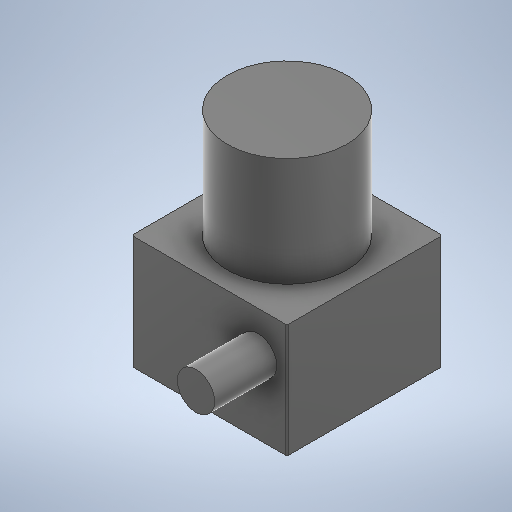
# Autodesk Inventor part: RE38S-600Z-1M-no-end
Saved by Autodesk Inventor 2026.2 (Build 302298010, 298A)
## iProperties
Created: 2026-05-12
Part Number: RE38S-600Z-1M-no-end
Material: ABS Plastic
Document SubType Name: Modeling
Designer: chanh
Density: 1.06 g/cm^3
Appearance: Smooth - White
Author: chanh
Autodesk Inventor part; units mm, degrees
ref_plane "YZ Plane" through (0, 0, 0) normal (1, 0, 0) x (0, 1, 0)
ref_plane "XZ Plane" through (0, 0, 0) normal (0, 1, 0) x (-1, 0, 0)
sketch "Sketch1" plane through (0, 0, 0) normal (0, 1, 0) x (-1, 0, 0)
  line L0 (-25, 25) -> (25, 25)
  line L1 (25, 25) -> (25, -25)
  line L2 (25, -25) -> (-25, -25)
  line L3 (-25, -25) -> (-25, 25)
  line L4 (-25, 25) -> (25, -25) construction
  line L5 (25, 25) -> (-25, -25) construction
  point P0 (0, 0)
  dimension "d0" = 50
  dimension "d1" = 50
  constraints: 12 end point, 2 midpoint, 2 parallel, 1 horizontal, 1 perpendicular
  measures "d0" distance of L1.end L2.end
  measures "d1" distance of L0.end L1.end
extrude "Extrusion1" add sketch "Sketch1" along normal blind 36.5
sketch "Sketch2" plane through (-25, 0, 25) normal (0, 0, 1) x (1, 0, 0)
  line L0 (0, 0) -> (50, 0) projected
  line L1 (50, 0) -> (50, 36.5) projected
  line L2 (0, 36.5) -> (50, 36.5) projected
  line L3 (0, 0) -> (0, 36.5) projected
  circle A0 centre (40.7, 23.5) radius 6
  line L4 (25, 0) -> (25, 36.5) construction
  dimension "d4" = 15.7
  dimension "d5" = 13
  dimension "d6" = 12
  constraints: 2 end point, 1 centre point, 1 midpoint
  measures "d4" distance from line of A0.centre L4
  measures "d5" distance from line of L2 A0.centre
  measures "d6" diameter of A0
extrude "Extrusion2" add sketch "Sketch2" along normal blind 20 contours A0
sketch "Sketch4" plane through (0, 36.5, 0) normal (0, 1, 0) x (1, 0, 0)
  circle A0 centre (0, 0) radius 19.25
  dimension "d12" = 38.5
  constraints: 1 centre point, 1 coincident
  measures "d12" diameter of A0
extrude "Extrusion4" add sketch "Sketch4" along normal blind 35
sketch "Sketch7" plane through (25, 0, -25) normal (0, 0, -1) x (-1, 0, 0)
  line L0 (0, 0) -> (50, 0) projected
  line L1 (50, 0) -> (50, 36.5) projected
  line L2 (0, 36.5) -> (50, 36.5) projected
  line L3 (0, 0) -> (0, 36.5) projected
  line L4 (12.5, 22.5) -> (37.5, 22.5) construction
  point P0 (25, 0)
  point P1 (25, 22.5)
  point P2 (25, 0)
  dimension "d22" = 25
  dimension "d23" = 22.5
  constraints: 2 end point, 2 midpoint, 1 horizontal, 1 vertical alignment
  measures "d22" distance of L4.end L4.start
  measures "d23" distance between parallel lines of L4 L0
hole "Hole2" at (12.5, 22.5, -25) at (-12.5, 22.5, -25) direction (0, 0, 1) diameter 4.134 depth 8 thread size "M5x0.8" class "6H" standard "ISO Metric profile"
sketch "Sketch9" plane through (-25, 0, -25) normal (-1, 0, 0) x (0, 0, 1)
  line L0 (0, 0) -> (50, 0) projected
  line L1 (50, 0) -> (50, 36.5) projected
  line L2 (0, 36.5) -> (50, 36.5) projected
  line L3 (0, 0) -> (0, 36.5) projected
  line L4 (12.5, 22.5) -> (37.5, 22.5) construction
  point P0 (25, 0)
  point P1 (25, 22.5)
  point P2 (25, 0)
  dimension "d38" = 25
  dimension "d39" = 22.5
  constraints: 2 end point, 2 midpoint, 1 horizontal, 1 vertical alignment
  measures "d38" distance of L4.end L4.start
  measures "d39" distance between parallel lines of L4 L0
hole "Hole3" at (-25, 22.5, -12.5) at (-25, 22.5, 12.5) direction (1, 0, 0) diameter 4.134 depth 8 thread size "M5x0.8" class "6H" standard "ISO Metric profile"
chamfer "Chamfer1" distance 0.5 angle 45 4 edges at (25, 18.25, 25) (-25, 18.25, 25) (25, 18.25, -25) (-25, 18.25, -25)
sketch "Sketch10" plane through (15.7, 23.5, 45) normal (0, 0, 1) x (1, 0, 0)
  circle A0 centre (0, 0) radius 6 projected
  point P0 (-15.7, -23.5)
ref_plane "Work Plane4" through (15.7, 23.5, 45) normal (0, -1, 0) x (1, 0, 0)
body "Solid1"
